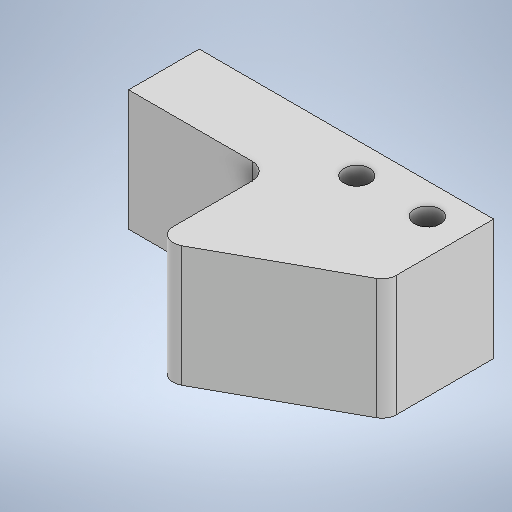
# Autodesk Inventor part: mogo aligner
Saved by Autodesk Inventor 2025.2 (Build 292293000, 293)
## iProperties
Created: 2024-12-10
Part Number: mogo aligner
Material: Generic
Document SubType Name: Modeling
Designer: hmath
Density: 1 g/cm^3
Appearance: Default
Author: hmath
Autodesk Inventor part; units mm, degrees
ref_plane "YZ Plane" through (0, 0, 0) normal (1, 0, 0) x (0, 1, 0)
ref_plane "XZ Plane" through (0, 0, 0) normal (0, 1, 0) x (-1, 0, 0)
ref_plane "XY Plane" through (0, 0, 0) normal (0, 0, 1) x (1, 0, 0)
sketch "Sketch1" plane through (0, 0, 0) normal (0, 0, 1) x (1, 0, 0)
  line L0 (0, 0) -> (52.959, 0)
  line L1 (52.959, 0) -> (52.959, 21.717)
  line L2 (52.959, 21.717) -> (0, 21.717)
  line L3 (0, 21.717) -> (0, 0)
  dimension "d0" = 52.959
  dimension "d1" = 21.717
  constraints: 8 end point, 2 parallel, 1 horizontal, 1 perpendicular
  measures "d0" distance of L1.end L2.end
  measures "d1" distance of L0.end L1.end
extrude "Extrusion1" add sketch "Sketch1" along normal blind 12.7
sketch "Sketch3" plane through (0, 21.717, 0) normal (0, 1, 0) x (1, 0, 0)
  line L0 (52.959, -12.7) -> (0, -12.7) projected
  line L1 (52.959, -12.7) -> (25.3122, -12.7)
  line L2 (25.3122, -26.2939) -> (25.3122, -12.7)
  line L3 (25.3122, -26.2939) -> (25.3122, -34.29)
  line L4 (52.959, -12.7) -> (52.959, -19.05)
  line L5 (52.959, -19.05) -> (25.3122, -34.29)
  line L6 (25.3122, -34.29) -> (25.3122, -35.7538)
  point P0 (0, 0)
  dimension "d20" = 6.35
  dimension "d21" = 21.59
  constraints: 12 end point, 2 vertical, 1 parallel, 1 perpendicular, 1 point on line
  measures "d20" distance of L0.start L4.end
  measures "d21" distance of L3.end L1.end
extrude "Extrusion2" add sketch "Sketch3" against normal up to surface (21.717 mm away)
fillet "Fillet2" radius 3.1115 1 edges at (25.3122, 10.8585, 12.7)
sketch "Sketch4" plane through (0, 21.717, 0) normal (0, 1, 0) x (1, 0, 0)
  line L0 (52.959, 0) -> (52.959, -19.05) projected
  line L1 (52.959, 0) -> (52.959, -5.5626)
  line L2 (52.959, -5.5626) -> (46.609, -5.5626)
  circle A0 centre (46.609, -5.5626) radius 2.3241
  line L3 (52.959, 0) -> (0, 0) projected
  circle A1 centre (33.909, -5.5626) radius 2.3241
  circle A2 centre (21.209, -5.5626) radius 2.3241
  circle A3 centre (8.509, -5.5626) radius 2.3241
  circle A4 centre (-4.191, -5.5626) radius 2.3241
  point P0 (52.959, -11.0236)
  dimension "d8" = 6.35
  dimension "d9" = 4.6482
  dimension "d12" = 5.5626
  dimension "d15" = 12.7
  constraints: 5 centre point, 4 end point, 1 coincident, 1 horizontal, 1 perpendicular, 1 point on line, 8 other
  measures "d8" distance of L1.end L2.end
  measures "d9" diameter of A0
  measures "d12" distance between parallel lines of L3 L2
  measures "d15" distance of A0.centre A1.centre
extrude "Extrusion3" cut sketch "Sketch4" against normal through all contours A0 | A1
fillet "Fillet3" radius 2.54 2 edges at (25.3122, 10.8585, 34.29) (52.959, 10.8585, 19.05)
body "Solid1"
